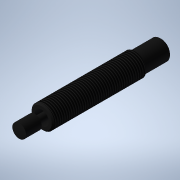
# Autodesk Inventor part: 548072 DYSW-7-10-Y1F---(SD_0)
Saved by Autodesk Inventor 2021 (Build 250183000, 183)
## iProperties
Created: 2026-04-25
Part Number: 548072 DYSW-7-10-Y1F---(SD_0)
Material: Generic
Catalog Web Link: www.3dfindit.com
Description: DYSW-(SD)-shock absorber
Vendor: FESTO
Document SubType Name: Modeling
Designer: psAdmin
Manufacturer: FESTO
Mass: 3.88747 g
Surface Area: 21.344 cm^2
Volume: 3.88747 cm^3
Density: 1 g/cm^3
Appearance: PSOLRGB-128-128-128
Category: PARTsolutions
Company: FESTO
Title: 548072 DYSW-7-10-Y1F
Author: Cadenas PARTsolutions
Comments: shock absorber
PSOL_IDENT_0: {$CADENAS_DATA/23d-libs/festo/parts/d/dysw/parts/dysw_sd.prj},202 {VTYP=3D},{NB=548072 DYSW-7-10-Y1F
PSOL_IDENT_1: ---(SD_0)},{LINA=548072 DYSW-7-10-Y1F},{NN=DYSW-(SD)},{DATE=07.03.2024 14:36:08},{GEOMDATE=07.03.202
PSOL_IDENT_2: 4 14:19:03},{VERSION=},{LINEID=30},{WBVAR=HUBST},{WBNUMERIC=HUBST}  {NB=548072 DYSW-7-10-Y1F---(SD_0
PSOL_IDENT_3: )},{LINA=548072 DYSW-7-10-Y1F},{KT=DUMMY},{TNR=548072},{TYP=DYSW-7-10-Y1F},{HUBST=0},{D1=M10x1},{D1N=
PSOL_IDENT_4: 10.000},{D1K=9.000},{D1PITCH=1.000},{D2=3.000},{D3=6.000},{D4=8.600},{L1=52.050},{L2=41.050},{L3=10.
PSOL_IDENT_5: 000},{L4=7.000},{B=3.500},{SW1=13.000},{SW2=3.000},{T=2.000},{NUTTNR=396998},{FDTDADPB=20.000}
NB: 548072 DYSW-7-10-Y1F---(SD_0)
NN: DYSW-(SD)
NT: shock absorber
NBSYN: $TNR. $TYP.---(SD_$HUBST.)
LINA: 548072 DYSW-7-10-Y1F
CATALOG: Festo
TNR: 548072
TYP: DYSW-7-10-Y1F
HUBST: 0
D1: M10x1
D1N: 10
D1K: 9
D1PITCH: 1
D2: 3
D3: 6
D4: 8.6
L1: 52.05
L2: 41.05
L3: 10
L4: 7
B: 3.5
SW1: 13
SW2: 3
T: 2
NUTTNR: 396998
FDTDADPB: 20
SUPPLIER: FESTO
ARTICLENO: 548072 DYSW-7-10-Y1F---(SD_0)
BOMINFO: 548072 DYSW-7-10-Y1F
CREATOR: CADENAS GmbH
Autodesk Inventor part; units mm, degrees
sketch "Skizze_1" plane through (0, 0, 0) normal (1, 0, 0) x (0, 1, 0)
  line L0 (0, -52.05) -> (0, 0)
  line L1 (0, -7) -> (3.1, -7)
  line L2 (3.1, -7) -> (3.1, 0)
  line L3 (3.1, 0) -> (4.3865, 0)
  line L4 (4.3865, 0) -> (5, -0.6135)
  line L5 (5, -0.6135) -> (5, -40.4365)
  line L6 (5, -40.4365) -> (4.3865, -41.05)
  line L7 (4.3865, -41.05) -> (4.3, -41.05)
  line L8 (4.3, -41.05) -> (4.3, -51.55)
  line L9 (4.3, -51.55) -> (3.8, -52.05)
  line L10 (3.8, -52.05) -> (0, -52.05)
  line L11 (0, -52.05) -> (0, -7)
  constraints: 24 end point
revolve "Revolution1" add sketch "Skizze_1" angle 360 about axis through (0, 0, -52.05) along (0, 0, -1)
thread "Thread1" size "M10x1" class "6g" standard "ISO Metric profile" full length
sketch "Skizze_3" plane through (0, 0, 0) normal (1, 0, 0) x (0, 1, 0)
  line L0 (0, -14) -> (0, 10)
  arc A0 (3, 9.8118) -> (0, 10) centre (0, -14) ccw
  line L1 (3, 9.8118) -> (3, 3)
  line L2 (3, 3) -> (1.5, 3)
  line L3 (1.5, 3) -> (1.5, -14)
  line L4 (1.5, -14) -> (0, -14)
  line L5 (0, -14) -> (0, 10)
  constraints: 12 end point, 2 point on circle, 1 centre point
revolve "Revolution2" add sketch "Skizze_3" angle 360 about axis through (0, 0, -14) along (0, 0, -1)
sketch "Skizze_4" plane through (0, 0, -52.05) normal (0, 0, -1) x (0, 1, 0)
  line L0 (-1.5, -0.866) -> (0, -1.7321)
  line L1 (0, -1.7321) -> (1.5, -0.866)
  line L2 (1.5, -0.866) -> (1.5, 0.866)
  line L3 (1.5, 0.866) -> (0, 1.7321)
  line L4 (0, 1.7321) -> (-1.5, 0.866)
  line L5 (-1.5, 0.866) -> (-1.5, -0.866)
  constraints: 12 end point
extrude "Extrusion1" cut sketch "Skizze_4" against normal blind 2
ref_plane "FDT_ANBAU_XY" through (0, 0, -1.5) normal (0, 0, -1) x (1, 0, 0)
ref_plane "FDT_ANBAU_YZ" through (0, 0, -1.5) normal (1, 0, 0) x (0, -1, 0)
ref_plane "FDT_ANBAU_ZX" through (0, 0, -1.5) normal (0, -1, 0) x (0, 0, -1)
ref_plane "FDT_NUT_XY" through (0, 0, -21.5) normal (0, 0, 1) x (1, 0, 0)
ref_plane "FDT_NUT_YZ" through (0, 0, -21.5) normal (1, 0, 0) x (0, 1, 0)
ref_plane "FDT_NUT_ZX" through (0, 0, -21.5) normal (0, 1, 0) x (0, 0, 1)
ref_plane "IP_DGSL_XY" through (0, 0, -52.05) normal (0, 0, -1) x (0, 1, 0)
ref_plane "IP_DGSL_YZ" through (0, 0, -52.05) normal (0, 1, 0) x (1, 0, 0)
ref_plane "IP_DGSL_ZX" through (0, 0, -52.05) normal (1, 0, 0) x (0, 0, -1)
ref_plane "NUT1_XY" through (0, 0, -17.025) normal (0, 0, 1) x (1, 0, 0)
ref_plane "NUT1_YZ" through (0, 0, -17.025) normal (1, 0, 0) x (0, 1, 0)
ref_plane "NUT1_ZX" through (0, 0, -17.025) normal (0, 1, 0) x (0, 0, 1)
ref_plane "NUT2_XY" through (0, 0, -24.025) normal (0, 0, 1) x (1, 0, 0)
ref_plane "NUT2_YZ" through (0, 0, -24.025) normal (1, 0, 0) x (0, 1, 0)
ref_plane "NUT2_ZX" through (0, 0, -24.025) normal (0, 1, 0) x (0, 0, 1)
body "Solid1"
